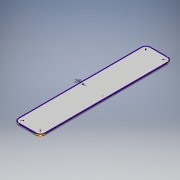
# Autodesk Inventor part: EtgSignModV2
Saved by Autodesk Inventor 2019 (Build 230136000, 136)
## iProperties
Created: 2018-10-30
Part Number: EtgSignModV2
Material: Generic
Document SubType Name: Modeling
Designer: Administrator
Density: 1 g/cm^3
Appearance: Default
Author: Administrator
Autodesk Inventor part; units mm, degrees
ref_plane "YZ Plane" through (0, 0, 0) normal (1, 0, 0) x (0, 1, 0)
ref_plane "XZ Plane" through (0, 0, 0) normal (0, 1, 0) x (-1, 0, 0)
ref_plane "XY Plane" through (0, 0, 0) normal (0, 0, 1) x (1, 0, 0)
sketch "Sketch1" plane through (0, 0, 0) normal (0, 1, 0) x (-1, 0, 0)
  line L0 (53.975, 0) -> (250.825, 0)
  line L1 (304.8, -53.975) -> (304.8, -1470.025)
  line L2 (250.825, -1524) -> (53.975, -1524)
  line L3 (0, -1470.025) -> (0, -53.975)
  circle A0 centre (263.525, -41.275) radius 5.5563
  circle A1 centre (263.525, -762) radius 5.5563
  circle A2 centre (263.525, -1482.725) radius 5.5563
  circle A3 centre (41.275, -41.275) radius 5.5563
  circle A4 centre (41.275, -762) radius 5.5563
  circle A5 centre (41.275, -1482.725) radius 5.5563
  arc A6 (304.8, -53.975) -> (250.825, 0) centre (250.825, -53.975) ccw
  arc A7 (0, -1470.025) -> (53.975, -1524) centre (53.975, -1470.025) ccw
  arc A8 (250.825, -1524) -> (304.8, -1470.025) centre (250.825, -1470.025) ccw
  arc A9 (53.975, 0) -> (0, -53.975) centre (53.975, -53.975) ccw
  point P0 (0, 0)
  point P1 (304.8, -1524)
  point P2 (0, -1524)
  dimension "d0" = 304.8
  dimension "d1" = 1524
  dimension "d2" = 11.1125
  dimension "d5" = 720.725
  dimension "d8" = 222.25
  dimension "d11" = 41.275
  dimension "d12" = 41.275
  dimension "d13" = 53.975
  constraints: 10 centre point, 8 end point, 8 point on circle, 8 tangent, 6 point on line, 3 equal radius, 2 horizontal, 2 parallel, 1 perpendicular, 1 vertical, 10 other
  measures "d0" distance of point (304.8, -1524) point (0, -1524)
  measures "d1" distance between parallel lines of L2 L0
  measures "d2" diameter of A0
  measures "d5" distance of A0.centre A1.centre
  measures "d8" distance of A0.centre A3.centre
  measures "d11" distance from line of L0 A0.centre
  measures "d12" distance from line of L1 A0.centre
  measures "d13" radius of A6
extrude "Extrusion1" add sketch "Sketch1" along normal blind 22.225
ref_plane "Work Plane3" through (0, 17.4625, 0) normal (0, 1, 0) x (1, 0, 0)
sketch "Sketch2" plane through (0, 17.4625, 0) normal (0, 1, 0) x (1, 0, 0)
  circle A0 centre (-41.275, 1482.725) radius 5.5562 projected
  circle A1 centre (-41.275, 762) radius 5.5562 projected
  circle A2 centre (-41.275, 41.275) radius 5.5562 projected
  circle A3 centre (-263.525, 1482.725) radius 5.5562 projected
  circle A4 centre (-263.525, 762) radius 5.5562 projected
  circle A5 centre (-263.525, 41.275) radius 5.5562 projected
  line L0 (-250.825, 0) -> (-53.975, 0) projected
  arc A6 (-53.975, 0) -> (0, 53.975) centre (-53.975, 53.975) ccw projected
  line L1 (0, 53.975) -> (0, 1470.025) projected
  arc A7 (0, 1470.025) -> (-53.975, 1524) centre (-53.975, 1470.025) ccw projected
  line L2 (-53.975, 1524) -> (-250.825, 1524) projected
  arc A8 (-250.825, 1524) -> (-304.8, 1470.025) centre (-250.825, 1470.025) ccw projected
  line L3 (-304.8, 1470.025) -> (-304.8, 53.975) projected
  arc A9 (-304.8, 53.975) -> (-250.825, 0) centre (-250.825, 53.975) ccw projected
  line L4 (0, 53.975) -> (0, 1470.025)
  arc A10 (-250.825, 1524) -> (-304.8, 1470.025) centre (-250.825, 1470.025) ccw projected
  line L5 (-53.975, 1524) -> (-250.825, 1524)
  line L6 (-304.8, 1470.025) -> (-304.8, 53.975) projected
  line L7 (-304.8, 1470.025) -> (-304.8, 53.975)
  line L8 (-250.825, 0) -> (-53.975, 0)
  point P0 (0, 0)
  constraints: 8 end point, 2 horizontal, 2 vertical, 1 tangent
ref_plane "Work Plane4" through (0, 4.7625, 0) normal (0, -1, 0) x (1, 0, 0)
sketch "Sketch3" plane through (0, 4.7625, 0) normal (0, -1, 0) x (1, 0, 0)
  circle A0 centre (-41.275, -1482.725) radius 5.5562 projected
  circle A1 centre (-41.275, -762) radius 5.5562 projected
  circle A2 centre (-41.275, -41.275) radius 5.5562 projected
  circle A3 centre (-263.525, -1482.725) radius 5.5562 projected
  circle A4 centre (-263.525, -762) radius 5.5562 projected
  circle A5 centre (-263.525, -41.275) radius 5.5562 projected
  line L0 (-250.825, 0) -> (-53.975, 0) projected
  arc A6 (0, -53.975) -> (-53.975, 0) centre (-53.975, -53.975) ccw projected
  line L1 (0, -53.975) -> (0, -1470.025) projected
  arc A7 (-53.975, -1524) -> (0, -1470.025) centre (-53.975, -1470.025) ccw projected
  line L2 (-53.975, -1524) -> (-250.825, -1524) projected
  arc A8 (-304.8, -1470.025) -> (-250.825, -1524) centre (-250.825, -1470.025) ccw projected
  line L3 (-304.8, -1470.025) -> (-304.8, -53.975) projected
  arc A9 (-250.825, 0) -> (-304.8, -53.975) centre (-250.825, -53.975) ccw projected
  line L4 (-299.72, -53.975) -> (-299.72, -1470.025)
  arc A10 (-299.72, -1470.025) -> (-250.825, -1518.92) centre (-250.825, -1470.025) ccw
  line L5 (-250.825, -1518.92) -> (-53.975, -1518.92)
  arc A11 (-53.975, -1518.92) -> (-5.08, -1470.025) centre (-53.975, -1470.025) ccw
  line L6 (-5.08, -1470.025) -> (-5.08, -53.975)
  arc A12 (-5.08, -53.975) -> (-53.975, -5.08) centre (-53.975, -53.975) ccw
  line L7 (-53.975, -5.08) -> (-250.825, -5.08)
  arc A13 (-250.825, -5.08) -> (-299.72, -53.975) centre (-250.825, -53.975) ccw
  point P0 (0, 0)
  dimension "d26" = 5.08
  constraints: 8 end point, 8 point on circle, 4 centre point, 7 other
  measures "d26" distance between parallel lines of L3 L4
sketch "Sketch8" plane through (0, 22.225, 0) normal (0, 1, 0) x (1, 0, 0)
  arc A0 (-53.975, 0) -> (0, 53.975) centre (-53.975, 53.975) ccw projected
  line L0 (-250.825, 0) -> (-53.975, 0) projected
  line L1 (-53.975, 0) -> (-250.825, 0)
  arc A1 (-304.8, 53.975) -> (-250.825, 0) centre (-250.825, 53.975) ccw projected
  arc A2 (-250.825, 1524) -> (-304.8, 1470.025) centre (-250.825, 1470.025) ccw projected
  line L2 (-304.8, 53.975) -> (-304.8, 1470.025)
  line L3 (-53.975, 1524) -> (-250.825, 1524) projected
  line L4 (-250.825, 1524) -> (-53.975, 1524)
  arc A3 (0, 1470.025) -> (-53.975, 1524) centre (-53.975, 1470.025) ccw projected
  line L5 (0, 1470.025) -> (0, 53.975)
  arc A4 (-53.975, 0) -> (0, 53.975) centre (-53.975, 53.975) ccw
  arc A5 (-304.8, 53.975) -> (-250.825, 0) centre (-250.825, 53.975) ccw
  arc A6 (-250.825, 1524) -> (-304.8, 1470.025) centre (-250.825, 1470.025) ccw
  arc A7 (0, 1470.025) -> (-53.975, 1524) centre (-53.975, 1470.025) ccw
  line L6 (-299.72, 1470.025) -> (-299.72, 53.975)
  arc A8 (-299.72, 53.975) -> (-250.825, 5.08) centre (-250.825, 53.975) ccw
  line L7 (-250.825, 5.08) -> (-53.975, 5.08)
  arc A9 (-53.975, 5.08) -> (-5.08, 53.975) centre (-53.975, 53.975) ccw
  line L8 (-5.08, 53.975) -> (-5.08, 1470.025)
  arc A10 (-5.08, 1470.025) -> (-53.975, 1518.92) centre (-53.975, 1470.025) ccw
  line L9 (-53.975, 1518.92) -> (-250.825, 1518.92)
  arc A11 (-250.825, 1518.92) -> (-299.72, 1470.025) centre (-250.825, 1470.025) ccw
  point P0 (0, 0)
  dimension "d25" = 5.08
  constraints: 16 end point, 16 point on circle, 9 tangent, 8 centre point, 2 horizontal, 2 vertical, 7 other
  measures "d25" distance between parallel lines of L2 L6
extrude "Extrusion2" cut sketch "Sketch3" against normal blind 12.7 contours L0 A6 L1 A7 L2 A8 L3 A9
body "Solid1"
